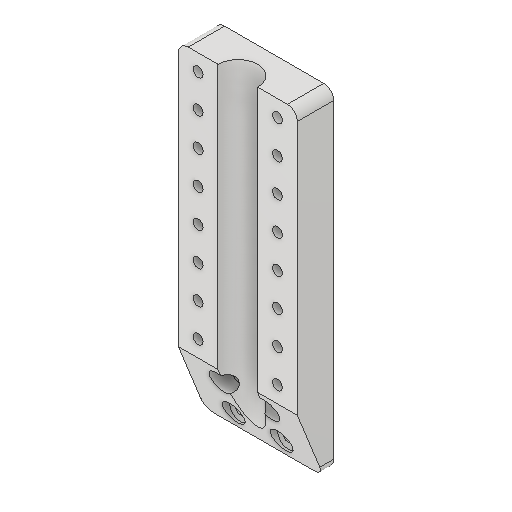
# Autodesk Inventor part: 3DP_PLA_X_axis_carriage_laser_mount
Saved by Autodesk Inventor 2025 (Build 290162010, 162A)
## iProperties
Created: 2018-08-01
Part Number: 3DP_PLA_X_axis_carriage_laser_mount
Material: ABS Plastic
Document SubType Name: Modeling
Designer: Andrzej
Density: 1.06 g/cm^3
Appearance: Smooth - White
Author: Andrzej
Autodesk Inventor part; units mm, degrees
ref_plane "YZ Plane" through (0, 0, 0) normal (1, 0, 0) x (0, 1, 0)
ref_plane "XZ Plane" through (0, 0, 0) normal (0, 1, 0) x (-1, 0, 0)
ref_plane "XY Plane" through (0, 0, 0) normal (0, 0, 1) x (1, 0, 0)
sketch "Sketch1" plane through (0, 0, 0) normal (0, 0, 1) x (1, 0, 0)
  line L0 (-8.7244, 5.8803) -> (27.2756, 5.8803)
  line L1 (27.2756, 5.8803) -> (27.2756, -4.1197)
  line L2 (27.2756, -4.1197) -> (-8.7244, -4.1197)
  line L3 (-8.7244, -4.1197) -> (-8.7244, 5.8803)
  point P0 (0, 0)
  point P1 (-2.7244, 0.8803)
  point P2 (21.2756, 0.8803)
  dimension "d0" = 36
  dimension "d1" = 24
  dimension "d2" = 6
  dimension "d3" = 10
  dimension "d4" = 5
  constraints: 8 end point, 2 parallel, 1 horizontal, 1 horizontal alignment, 1 perpendicular
  measures "d0" distance of L1.end L2.end
  measures "d1" distance of point (21.276, 0.88) point (-2.724, 0.88)
  measures "d2" distance from line of L3 point (-2.724, 0.88)
  measures "d3" distance between parallel lines of L2 L0
  measures "d4" distance from line of L0 point (-2.724, 0.88)
extrude "Extrusion1" add sketch "Sketch1" along normal blind 8
hole "Hole1" at (-2.7244, 0.8803, 0) at (21.2756, 0.8803, 0) direction (0, 0, 1) diameter 3 end through all
sketch "Sketch2" plane through (-8.7244, 5.8803, 0) normal (0, 1, 0) x (1, 0, 0)
  line L0 (0, 0) -> (36, 0) projected
  line L1 (0, 0) -> (0, -8) projected
  line L2 (36, -8) -> (0, -8) projected
  line L3 (36, 0) -> (36, -8) projected
  line L4 (0, -8) -> (36, -8) projected
  circle A0 centre (18, -8) radius 6
  point P0 (8.7244, 0)
  dimension "d14" = 12
  dimension "d15" = 36
  dimension "d16" = 18
  constraints: 1 centre point, 1 midpoint
  measures "d14" diameter of A0
  measures "d15" distance between parallel lines of L3 L1
  measures "d16" distance from line of L1 A0.centre
extrude "Extrusion2" cut sketch "Sketch2" against normal through all contours A0 L2 | L2 A0
pattern_linear "Rectangular Pattern1" count 8 spacing 10 along (0, 1, 0) of "Extrusion1", "Extrusion2", "Hole1"
sketch "Sketch3" plane through (0, 0, 0) normal (0, 0, -1) x (-1, 0, 0)
  circle A0 centre (-21.2756, 60.8803) radius 1.5 projected
  circle A1 centre (2.7244, 60.8803) radius 1.5 projected
  circle A2 centre (-21.2756, 40.8803) radius 1.5 projected
  circle A3 centre (2.7244, 40.8803) radius 1.5 projected
  circle A4 centre (-21.2756, 20.8803) radius 1.5 projected
  circle A5 centre (2.7244, 20.8803) radius 1.5 projected
  circle A6 centre (-21.2756, 10.8803) radius 1.5 projected
  circle A7 centre (2.7244, 10.8803) radius 1.5 projected
  circle A8 centre (2.7244, 30.8803) radius 1.5 projected
  circle A9 centre (-21.2756, 30.8803) radius 1.5 projected
  circle A10 centre (2.7244, 50.8803) radius 1.5 projected
  circle A11 centre (-21.2756, 50.8803) radius 1.5 projected
  circle A12 centre (2.7244, 70.8803) radius 1.5 projected
  circle A13 centre (-21.2756, 70.8803) radius 1.5 projected
  circle A14 centre (2.7244, 0.8803) radius 1.5 projected
  circle A15 centre (-21.2756, 0.8803) radius 1.5 projected
  line L0 (-27.2756, 75.8803) -> (-27.2756, -4.1197) projected
  line L1 (-27.2756, -4.1197) -> (8.7244, -4.1197) projected
  line L2 (8.7244, -4.1197) -> (8.7244, 75.8803) projected
  line L3 (-27.2756, -4.1197) -> (8.7244, -4.1197)
  line L4 (8.7244, -4.1197) -> (8.7244, -24.1197)
  line L5 (8.7244, -24.1197) -> (-27.2756, -24.1197)
  line L6 (-27.2756, -24.1197) -> (-27.2756, -4.1197)
  line L7 (8.7244, 75.8803) -> (-27.2756, 75.8803) projected
  point P0 (0, 0)
  point P1 (-16.5256, -9.1197)
  point P2 (-2.0256, -9.1197)
  point P3 (-16.5256, -19.1197)
  point P4 (-2.0256, -19.1197)
  dimension "d25" = 20
  dimension "d26" = 36
  dimension "d27" = 10.75
  dimension "d28" = 10.75
  dimension "d29" = 5
  dimension "d30" = 5
  constraints: 8 end point, 2 horizontal alignment, 2 parallel, 2 vertical alignment, 1 horizontal, 1 perpendicular
  measures "d25" distance of L3.end L4.end
  measures "d26" distance of L4.end L5.end
  measures "d27" distance from line of L6 point (-16.526, -19.12)
  measures "d28" distance from line of L4 point (-2.026, -19.12)
  measures "d29" distance from line of L5 point (-16.526, -19.12)
  measures "d30" distance from line of L1 point (-16.526, -9.12)
extrude "Extrusion3" add sketch "Sketch3" along normal blind 3
chamfer "Chamfer2" distance 20 distance2 8 1 edges at (9.2756, -4.1197, 0) measured on face at (9.2756, -4.6197, 0)
hole "Hole2" at (16.5256, -9.1197, 0) at (2.0256, -9.1197, 0) at (16.5256, -19.1197, 0) at (2.0256, -19.1197, 0) direction (0, 0, 1) diameter 3 end through all both
hole "Hole3" at (16.5256, -19.1197, 0) at (2.0256, -19.1197, 0) at (2.0256, -9.1197, 0) at (16.5256, -9.1197, 0) direction (0, 0, 1) diameter 6.5 end through all
fillet "Fillet1" radius 3 4 edges at (-8.7244, -24.1197, -1.5) (27.2756, -24.1197, -1.5) (-8.7244, 75.8803, 2.5) (27.2756, 75.8803, 2.5)
equation "\"d2\" = -0.5 * d1 + 0.5 * d0"
equation "\"d16\" = 0.5 * d15"
equation "\"d28\" = d27"
body "Solid1"
